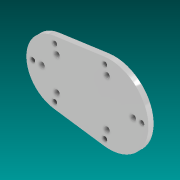
# Autodesk Inventor part: onderkantBasegefreesd
Saved by Autodesk Inventor 2020.2 (Build 242310000, 310)
## iProperties
Created: 2020-05-15
Part Number: onderkantBasegefreesd
Material: Aluminum 6061
Document SubType Name: Modeling
Designer: Svend
Density: 2.7 g/cm^3
Appearance: Aluminum - Polished
Author: Svend
Autodesk Inventor part; units mm, degrees
ref_plane "YZ Plane" through (0, 0, 0) normal (1, 0, 0) x (0, 1, 0)
ref_plane "XZ Plane" through (0, 0, 0) normal (0, 1, 0) x (-1, 0, 0)
ref_plane "XY Plane" through (0, 0, 0) normal (0, 0, 1) x (1, 0, 0)
sketch "Sketch1" plane through (0, 0, 0) normal (0, 0, 1) x (1, 0, 0)
  arc A0 (-5.9149, 42.0864) -> (-5.9149, -42.0864) centre (0, 0) ccw
  arc A1 (92.2885, -55.888) -> (92.2885, 55.888) centre (100.143, 0) ccw
  line L0 (-42.5, 0) -> (156.5802, 0)
  line L1 (92.2885, 55.888) -> (-5.9149, 42.0864)
  line L2 (-5.9149, -42.0864) -> (92.2885, -55.888)
  line L3 (-3.1314, 22.281) -> (95.0719, 36.0826)
  arc A2 (95.0719, -36.0826) -> (95.0719, 36.0826) centre (100.143, 0) ccw
  line L4 (95.0719, -36.0826) -> (-3.1314, -22.281)
  arc A3 (-3.1314, 22.281) -> (-3.1314, -22.281) centre (0, 0) ccw
  circle A4 centre (100.143, 0) radius 11
  line L5 (89.505, -75.6933) -> (-8.6983, -61.8918)
  arc A5 (-8.6983, 61.8918) -> (-8.6983, -61.8918) centre (0, 0) ccw
  line L6 (-8.6983, 61.8918) -> (89.505, 75.6933)
  arc A6 (89.505, -75.6933) -> (89.505, 75.6933) centre (100.143, 0) ccw
  point P0 (146.5802, 0)
  point P1 (95.0719, 46.1809)
  point P2 (95.0719, -46.1809)
  point P3 (-32.5, 0)
  point P4 (-3.1314, 32.3793)
  point P5 (-3.1314, -32.3793)
  dimension "d0" = 85
  dimension "d1" = 100.143
  dimension "d2" = 8
  dimension "d3" = 20
  dimension "d4" = 10
  dimension "d5" = 10
  dimension "d6" = 10
  dimension "d7" = 10
  dimension "d8" = 10
  dimension "d9" = 10
  dimension "d22" = 22
  dimension "d26" = 20
  constraints: 14 end point, 14 point on circle, 7 centre point, 4 tangent, 4 vertical alignment, 3 point on line, 2 coincident, 2 horizontal alignment, 1 horizontal, 6 other
  measures "d0" diameter of A0
  measures "d1" distance of A0.centre A1.centre
  measures "d2" angle of L0 L1
  measures "d3" distance between parallel lines of L1 L3
  measures "d4" distance from line of point (-3.131, -32.379) L4
  measures "d5" distance of L0.end point (146.58, 0)
  measures "d6" distance from line of L3 point (95.072, 46.181)
  measures "d7" distance from line of L3 point (-3.131, 32.379)
  measures "d8" distance from line of point (95.072, -46.181) L4
  measures "d9" distance of L0.start point (-32.5, 0)
  measures "d22" diameter of A4
  measures "d26" distance between parallel lines of L2 L5
extrude "Extrusion1" add sketch "Sketch1" along normal blind 10 contours L1 A1 L0 A2 L3 A3 A0 | L0 A3 L4 A2 A1 L2 A0 | A3 L3 A2 L0 A4 | L0 A4 A2 L4 A3 | L5 A5 L6 A6
sketch "Sketch4" plane through (0, 0, 10) normal (0, 0, 1) x (1, 0, 0)
  circle A0 centre (100.143, 0) radius 11.5 projected
  point P0 (0, 0)
extrude "Extrusion4" add sketch "Sketch4" against normal blind 2
hole "Hole3" at (146.5802, 0, 0) at (95.0719, 46.1809, 0) at (95.0719, -46.1809, 0) at (-32.5, 0, 0) at (-3.1314, 32.3793, 0) at (-3.1314, -32.3793, 0) direction (0, 0, 1) diameter 5.2 end through all
sketch "Sketch8" plane through (0, 0, 0) normal (0, 0, -1) x (-1, 0, 0)
  circle A0 centre (6.9587, -49.5134) radius 4.5
  circle A1 centre (-164.0802, 0) radius 4.5
  circle A2 centre (6.9587, 49.5134) radius 4.5
  circle A3 centre (-91.2447, 63.315) radius 4.5
  circle A4 centre (-91.2447, -63.315) radius 4.5
  circle A5 centre (50, 0) radius 4.5
  line L0 (8.6983, -61.8918) -> (-89.505, -75.6933)
  arc A6 (8.6983, -61.8918) -> (8.6983, 61.8918) centre (0, 0) ccw
  line L1 (-89.505, 75.6933) -> (8.6983, 61.8918)
  arc A7 (-89.505, 75.6933) -> (-89.505, -75.6933) centre (-100.143, 0) ccw
  circle A8 centre (32.5, 0) radius 2.067
  circle A9 centre (3.1314, 32.3793) radius 2.067
  circle A10 centre (-95.0719, 46.1809) radius 2.067
  circle A11 centre (-146.5802, 0) radius 2.067
  arc A12 (-94.3761, 41.0339) -> (-94.3761, -41.0339) centre (-100.143, 0) ccw
  line L2 (3.8273, 27.2324) -> (-94.3761, 41.0339)
  arc A13 (3.8273, -27.2324) -> (3.8273, 27.2324) centre (0, 0) ccw
  line L3 (-94.3761, -41.0339) -> (3.8273, -27.2324)
  circle A14 centre (-95.0719, -46.1809) radius 2.067
  circle A15 centre (3.1314, -32.3793) radius 2.067
  circle A16 centre (3.1314, 32.3793) radius 2.6 projected
  circle A17 centre (-95.0719, -46.1809) radius 2.6 projected
  circle A18 centre (-146.5802, 0) radius 2.6 projected
  circle A19 centre (-95.0719, 46.1809) radius 2.6 projected
  circle A20 centre (32.5, 0) radius 2.6 projected
  circle A21 centre (3.1314, -32.3793) radius 2.6 projected
  line L4 (-89.505, 75.6933) -> (8.6983, 61.8918) projected
  arc A22 (-89.505, 75.6933) -> (-89.505, -75.6933) centre (-100.143, 0) ccw projected
  line L5 (8.6983, -61.8918) -> (-89.505, -75.6933) projected
  arc A23 (8.6983, -61.8918) -> (8.6983, 61.8918) centre (0, 0) ccw projected
  constraints: 16 centre point, 8 end point, 8 point on circle, 1 coincident
hole "Hole6" at (164.0802, 0, 0) at (91.2447, -63.315, 0) at (-6.9587, -49.5134, 0) at (-50, 0, 0) at (-6.9587, 49.5134, 0) at (91.2447, 63.315, 0) direction (0, 0, 1) diameter 9 depth 40 tip angle 118 clearance for "Hex Head Cap Screw ISO 24017" size "M8" standard "ISO"
chamfer "Chamfer6" distance 3.5 angle 45 6 edges at (95.0719, 43.5809, 10) (146.5802, -2.6, 10) (95.0719, -48.7809, 10) (-3.1314, -34.9793, 10) (-32.5, -2.6, 10) (-3.1314, 29.7793, 10)
equation "\"d4\" = d7"
equation "\"d5\" = d8"
equation "\"d6\" = d7"
equation "\"d8\" = d7"
equation "\"d9\" = d4"
body "Solid1"
